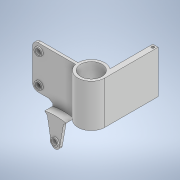
# Autodesk Inventor part: top_frame
Saved by Autodesk Inventor 2020 (Build 240168000, 168)
## iProperties
Created: 2020-03-09
Part Number: top_frame
Material: Generic
Document SubType Name: Modeling
Designer: xXxMrMayhemxXx
Density: 1 g/cm^3
Appearance: Default
Author: xXxMrMayhemxXx
Autodesk Inventor part; units mm, degrees
ref_plane "XZ Plane" through (0, 0, 0) normal (0, 1, 0) x (-1, 0, 0)
sketch "Sketch1" plane through (0, 0, 0) normal (0, 1, 0) x (-1, 0, 0)
  circle A0 centre (0, 0) radius 2
  circle A1 centre (0, 0) radius 2.5
  dimension "d0" = 4
  dimension "d1" = 5
  constraints: 2 centre point, 2 coincident
  measures "d0" diameter of A0
  measures "d1" diameter of A1
extrude "Extrusion1" add sketch "Sketch1" against normal blind 8
ref_plane "Work Plane2" through (0, 0, 0.5) normal (0, 0, 1) x (1, 0, 0)
sketch "Sketch3" plane through (0, 0, 0.5) normal (0, 0, 1) x (1, 0, 0)
  line L0 (-2.5, -8) -> (2.5, -8) projected
  line L1 (-2.5, 0) -> (-9.5, 0)
  line L2 (-10.5, -1) -> (-10.5, -7)
  line L3 (-9.5, -8) -> (-2.5, -8)
  arc A0 (-9.5, 0) -> (-10.5, -1) centre (-9.5, -1) ccw
  arc A1 (-10.5, -7) -> (-9.5, -8) centre (-9.5, -7) ccw
  line L4 (-2.5, -8) -> (-2.25, -8)
  line L5 (-2.25, -8) -> (-2.25, 0)
  line L6 (2.5, 0) -> (-2.5, 0) projected
  line L7 (-2.25, 0) -> (-2.5, 0)
  point P0 (0, 0)
  point P1 (-10.5, 0)
  dimension "d6" = 8
  dimension "d7" = 1
  dimension "d8" = 0.25
  constraints: 12 end point, 4 point on circle, 4 tangent, 3 point on line, 2 centre point, 2 parallel, 1 collinear, 1 equal radius, 1 horizontal
  measures "d6" distance of L1.start point (-10.5, 0)
  measures "d7" radius of A0
  measures "d8" distance of L3.end L4.end
extrude "Extrusion2" add sketch "Sketch3" against normal blind 0.5
sketch "Sketch4" plane through (0, 0, 0.5) normal (0, 0, 1) x (1, 0, 0)
  line L0 (-2.5, -8) -> (-9.5, -8) projected
  line L1 (-7.4495, -8) -> (-6.7247, -8.4184)
  line L2 (-6.7247, -8.4184) -> (-2.7247, -8.4184)
  line L3 (-2.5, -8) -> (2.5, -8) projected
  line L4 (-2.4495, -8) -> (-7.4495, -8)
  line L5 (-2, -8) -> (-2, 0) projected
  line L6 (-2, -8) -> (-2.7247, -8.4184)
  line L7 (-2, -8) -> (-7.4495, -8)
  point P0 (0, 0)
  dimension "d11" = 4
  dimension "d13" = 30
  dimension "d14" = 30
  constraints: 10 end point, 1 collinear, 1 horizontal, 1 point on line
  measures "d11" distance of L1.end L2.end
  measures "d13" angle of L0 L1
  measures "d14" angle of L0 L6
extrude "Extrusion3" add sketch "Sketch4" against normal up to surface (0.5 mm away)
sketch "Sketch5" plane through (0, 0, 0.5) normal (0, 0, 1) x (1, 0, 0)
  line L0 (-6.7247, -8.4184) -> (-2.7247, -8.4184) projected
  line L1 (-7.4495, -8) -> (-6.7247, -8.4184) projected
  line L2 (-2.7247, -8.4184) -> (-2, -8) projected
  line L3 (-2.7247, -8.4184) -> (-2.7247, -9.4184)
  line L4 (-2.7247, -9.4184) -> (-6.7247, -9.4184)
  line L5 (-6.7247, -9.4184) -> (-6.7247, -8.4184)
  point P0 (0, 0)
  dimension "d17" = 1
  constraints: 6 end point, 2 parallel, 1 horizontal, 1 perpendicular
  measures "d17" distance of L4.end L0.start
extrude "Extrusion4" add sketch "Sketch5" against normal up to surface (0.5 mm away)
chamfer "Chamfer1" distance 0.5 angle 45 2 edges at (-6.7247, -9.4184, 0.25) (-2.7247, -9.4184, 0.25)
sketch "Sketch6" plane through (0, 0, 0.5) normal (0, 0, 1) x (1, 0, 0)
  line L0 (-6.2247, -9.4184) -> (-3.2247, -9.4184) projected
  line L1 (-2.7247, -8.9184) -> (-2.7247, -8.4184) projected
  line L2 (-6.7247, -8.4184) -> (-6.7247, -8.9184) projected
  line L3 (-2.7247, -8.9184) -> (-3.2247, -9.4184) projected
  line L4 (-6.2247, -9.4184) -> (-6.7247, -8.9184) projected
  line L5 (-4.7247, -9.1684) -> (-4.7247, -9.4184)
  line L6 (-3.2247, -9.4184) -> (-6.2247, -9.4184) projected
  line L7 (-4.7247, -8.7164) -> (-4.7247, -5.942)
  line L8 (-6.7247, -8.9184) -> (-6.7247, -8.4184) projected
  arc A0 (-2.7247, -8.9184) -> (-6.7247, -8.9184) centre (-4.7247, -18.7164) ccw
  arc A1 (-3.2247, -9.4184) -> (-6.2247, -9.4184) centre (-4.7247, -13.7934) ccw
  point P0 (0, 0)
  dimension "d23" = 10
  constraints: 6 point on circle, 4 end point, 2 centre point, 1 midpoint
  measures "d23" radius of A0
extrude "Extrusion5" add sketch "Sketch6" along normal blind 1.5 contours L4 A0 L3 A1
sketch "Sketch7" plane through (0, 0, 0.5) normal (0, 0, 1) x (1, 0, 0)
  arc A0 (-3.2247, -9.4184) -> (-6.2247, -9.4184) centre (-4.7247, -13.7934) ccw projected
  line L0 (-6.2247, -9.4184) -> (-3.2247, -9.4184) projected
  point P0 (0, 0)
extrude "Extrusion6" cut sketch "Sketch7" against normal through all
sketch "Sketch8" plane through (0, 0, 2) normal (0, 0, 1) x (1, 0, 0)
  line L0 (-3.2247, -9.4184) -> (-2.7247, -8.9184) projected
  line L1 (-6.7247, -8.9184) -> (-6.2247, -9.4184) projected
  arc A0 (-3.2247, -9.4184) -> (-6.2247, -9.4184) centre (-4.7247, -13.7934) ccw projected
  line L2 (-3.2247, -9.4184) -> (-6.2247, -9.4184)
  point P0 (0, 0)
  constraints: 2 end point, 1 horizontal
extrude "Extrusion7" add sketch "Sketch8" against normal blind 0.5
sketch "Sketch9" plane through (-6.2247, -9.4184, 2) normal (0, -1, 0) x (1, 0, 0)
  line L0 (0, -0.5) -> (0, 0) projected
  line L1 (0, 0) -> (3, 0) projected
  line L2 (3, 0) -> (3, -0.5) projected
  line L3 (3, -0.5) -> (0, -0.5) projected
  point P0 (6.2247, -2)
extrude "Extrusion8" add sketch "Sketch9" along normal blind 4
sketch "Sketch10" plane through (0, 0, 2) normal (0, 0, 1) x (1, 0, 0)
  line L0 (-3.2247, -9.4184) -> (-3.2247, -13.4184) projected
  line L1 (-3.2247, -13.4184) -> (-6.2247, -13.4184) projected
  line L2 (-6.2247, -9.4184) -> (-6.2247, -13.4184) projected
  line L3 (-6.7247, -8.9184) -> (-6.2247, -9.4184) projected
  arc A0 (-2.7247, -8.9184) -> (-6.7247, -8.9184) centre (-4.7247, -18.7164) ccw projected
  line L4 (-3.2247, -9.4184) -> (-2.7247, -8.9184) projected
  line L5 (-3.2247, -9.4184) -> (-3.2247, -13.4184) projected
  line L6 (-3.2247, -9.4184) -> (-3.2247, -13.4184)
  line L7 (-3.2247, -13.4184) -> (-6.2247, -13.4184)
  line L8 (-6.2247, -9.4184) -> (-3.2247, -9.4184)
  line L9 (-6.2247, -9.4184) -> (-6.2247, -13.4184)
  line L10 (-3.2247, -9.4184) -> (-3.9369, -13.4573)
  line L11 (-5.5126, -13.4573) -> (-6.2247, -9.4184)
  arc A1 (-5.5126, -13.4573) -> (-3.9369, -13.4573) centre (-4.7247, -13.3183) ccw
  point P0 (0, 0)
  point P1 (-5.5194, -13.4184)
  point P2 (-3.9301, -13.4184)
  dimension "d32" = 10
  dimension "d33" = 10
  dimension "d34" = 0.8
  constraints: 12 end point, 2 perpendicular, 2 point on circle, 2 tangent, 2 vertical, 1 centre point
  measures "d32" angle of L0 L10
  measures "d33" angle of L2 L11
  measures "d34" radius of A1
extrude "Extrusion9" cut sketch "Sketch10" against normal through all contours L0 L1 L10 | L11 L1 L2
sketch "Sketch11" plane through (0, 0, 2) normal (0, 0, 1) x (1, 0, 0)
  line L0 (-3.9301, -13.4184) -> (-5.5194, -13.4184)
  line L1 (-3.9301, -13.4184) -> (-3.9369, -13.4573)
  line L2 (-5.5126, -13.4573) -> (-5.5194, -13.4184)
  arc A0 (-5.5126, -13.4573) -> (-3.9369, -13.4573) centre (-4.7247, -13.3183) ccw
  line L3 (-3.9301, -13.4184) -> (-5.5194, -13.4184) projected
  line L4 (-3.9301, -13.4184) -> (-5.5194, -13.4184)
  point P0 (0, 0)
  dimension "d39" = 0.8
  constraints: 8 end point, 2 point on circle, 2 point on line, 2 tangent, 1 centre point, 1 horizontal
  measures "d39" radius of A0
extrude "Extrusion10" add sketch "Sketch11" against normal up to surface (0.5 mm away)
sketch "Sketch12" plane through (0, 0, 2) normal (0, 0, 1) x (1, 0, 0)
  arc A0 (-5.5126, -13.4573) -> (-3.9369, -13.4573) centre (-4.7247, -13.3183) ccw projected
  line L0 (-4.7247, -14.1183) -> (-4.7247, -13.3183)
  line L1 (-4.7247, -13.3183) -> (-4.7247, -12.8683)
  circle A1 centre (-4.7247, -12.8683) radius 0.5
  point P0 (0, 0)
  dimension "d53" = 1
  dimension "d54" = 1.25
  constraints: 4 end point, 1 centre point, 1 coincident, 1 point on circle, 1 point on line, 1 vertical
  measures "d53" diameter of A1
  measures "d54" distance of L0.start L1.end
extrude "Extrusion11" cut sketch "Sketch12" against normal through all
sketch "Sketch13" plane through (0, 0, 0.5) normal (0, 0, 1) x (1, 0, 0)
  arc A0 (-10.5, -7) -> (-9.5, -8) centre (-9.5, -7) ccw projected
  arc A1 (-9.5, 0) -> (-10.5, -1) centre (-9.5, -1) ccw projected
  line L0 (-9.5, -1) -> (-9.25, -1.25)
  line L1 (-9.5, -1) -> (-4.2414, -1)
  line L2 (-2.4495, 0) -> (-9.5, 0) projected
  circle A2 centre (-9.25, -1.25) radius 0.5
  line L3 (-9.5, -7) -> (-4.4399, -7)
  line L4 (-9.5, -8) -> (-7.4495, -8) projected
  line L5 (-9.5, -7) -> (-9.25, -6.75)
  circle A3 centre (-9.25, -6.75) radius 0.5
  point P0 (0, 0)
  dimension "d45" = 45
  dimension "d46" = 1
  dimension "d47" = 0.25
  dimension "d48" = 45
  dimension "d49" = 1
  dimension "d50" = 0.25
  constraints: 8 end point, 2 centre point, 2 coincident, 2 horizontal, 2 parallel
  measures "d45" angle of L1 L0
  measures "d46" diameter of A2
  measures "d47" horizontal distance of L0.start L0.end
  measures "d48" angle of L5 L3
  measures "d49" diameter of A3
  measures "d50" horizontal distance of L3.start L5.end
extrude "Extrusion12" cut sketch "Sketch13" against normal through all
sketch "Sketch14" plane through (0, 0, 2) normal (0, 0, 1) x (1, 0, 0)
  circle A0 centre (-4.7247, -12.8683) radius 0.5 projected
  circle A1 centre (-4.7247, -12.8683) radius 0.75
  point P0 (0, 0)
  dimension "d55" = 1.5
  constraints: 1 centre point, 1 coincident
  measures "d55" diameter of A1
extrude "Extrusion13" add sketch "Sketch14" along normal blind 0.25
sketch "Sketch15" plane through (0, 0, 0.5) normal (0, 0, 1) x (1, 0, 0)
  circle A0 centre (-9.25, -1.25) radius 0.5 projected
  circle A1 centre (-9.25, -6.75) radius 0.5 projected
  circle A2 centre (-9.25, -1.25) radius 0.75
  circle A3 centre (-9.25, -6.75) radius 0.75
  point P0 (0, 0)
  dimension "d58" = 1.5
  dimension "d59" = 1.5
  constraints: 2 centre point, 2 coincident
  measures "d58" diameter of A2
  measures "d59" diameter of A3
extrude "Extrusion14" add sketch "Sketch15" along normal blind 0.25
ref_plane "Work Plane3" through (2, 0, 0) normal (1, 0, 0) x (0, 1, 0)
sketch "Sketch16" plane through (2, 0, 0) normal (1, 0, 0) x (0, 1, 0)
  line L0 (-8, 0) -> (-8, 0.5) projected
  line L1 (-8, 0) -> (-8, -10)
  line L2 (-8, -10) -> (0, -10)
  line L3 (0, -10) -> (0, 0)
  line L4 (-8, 0) -> (0, 0) projected
  dimension "d63" = 10
  constraints: 6 end point, 2 parallel, 2 perpendicular
  measures "d63" distance between parallel lines of L2 L4
extrude "Extrusion15" add sketch "Sketch16" along normal mid plane 1
sketch "Sketch17" plane through (0, 0, 0) normal (0, 1, 0) x (1, 0, 0)
  circle A0 centre (0, 0) radius 2
  circle A1 centre (0, 0) radius 2.5
  line L0 (1.5, 0) -> (1.5, 1.3229) projected
  line L1 (1.5, 0) -> (2, 0) projected
  line L2 (2.5, 10) -> (2.5, 0) projected
  dimension "d67" = 5
  dimension "d66" = 4
  constraints: 2 coincident, 1 centre point, 1 horizontal alignment, 1 other
  measures "d66" diameter of A0
extrude "Extrusion16" cut sketch "Sketch17" against normal through all contours L1 L0 A0 picked at (1.5908, 0.7499)
sketch "Sketch18" plane through (0, -8, 0) normal (0, -1, 0) x (1, 0, 0)
  line L0 (1.5, -10) -> (2.5, -10) projected
  line L1 (2.5, 0) -> (2.5, -10) projected
  line L2 (1.5, -10) -> (1.5, -2) projected
  line L3 (1.5, -9.5) -> (2.5, -9.5)
  line L4 (2, -10) -> (2, -9.5)
  circle A0 centre (2, -9.5) radius 0.25
  point P0 (0, 0)
  dimension "d70" = 0.5
  dimension "d71" = 0.5
  constraints: 4 end point, 2 midpoint, 2 point on line, 1 centre point, 1 coincident, 1 horizontal, 1 parallel
  measures "d70" diameter of A0
  measures "d71" distance of L4.start L4.end
extrude "Extrusion17" cut sketch "Sketch18" against normal through all contours A0 L3 L4 | L4 L3 A0 | A0 L3
body "Solid1"
